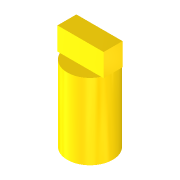
# Autodesk Inventor part: 00_laserpointer_red
Saved by Autodesk Inventor 2022 (Build 260153000, 153)
## iProperties
Created: 2023-04-20
Part Number: 00_laserpointer_red
Material: Generisch
Document SubType Name: Modeling
Designer: diederichbenedict
Density: 1 g/cm^3
Appearance: Glänzend - Gold
Author: diederichbenedict
Autodesk Inventor part; units mm, degrees
ref_plane "YZ Plane" through (0, 0, 0) normal (1, 0, 0) x (0, 1, 0)
ref_plane "XZ Plane" through (0, 0, 0) normal (0, 1, 0) x (-1, 0, 0)
ref_plane "XY Plane" through (0, 0, 0) normal (0, 0, 1) x (1, 0, 0)
sketch "Skizze1" plane through (0, 0, 0) normal (0, 1, 0) x (-1, 0, 0)
  circle A0 centre (0, 0) radius 3
  dimension "d0" = 6
  constraints: 1 centre point, 1 coincident
  measures "d0" diameter of A0
extrude "Extrusion1" add sketch "Skizze1" along normal blind 10
sketch "Skizze2" plane through (0, 10, 0) normal (0, 1, 0) x (1, 0, 0)
  line L0 (-3.05, -1.25) -> (3.05, -1.25)
  line L1 (3.05, -1.25) -> (3.05, 1.25)
  line L2 (3.05, 1.25) -> (-3.05, 1.25)
  line L3 (-3.05, 1.25) -> (-3.05, -1.25)
  line L4 (-3.05, -1.25) -> (3.05, 1.25) construction
  line L5 (3.05, -1.25) -> (-3.05, 1.25) construction
  point P0 (0, 0)
  dimension "d3" = 6.1
  dimension "d4" = 2.5
  constraints: 12 end point, 2 midpoint, 2 parallel, 1 horizontal, 1 perpendicular
  measures "d3" distance of L2.end L1.end
  measures "d4" distance of L1.end L0.end
extrude "Extrusion2" add sketch "Skizze2" along normal blind 3
